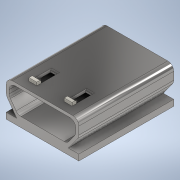
# Autodesk Inventor part: Port 3
Saved by Autodesk Inventor 2020 (Build 240168000, 168)
## iProperties
Created: 2022-11-24
Part Number: Port 3
Material: Generic
Document SubType Name: Modeling
Designer: DELL
Density: 1 g/cm^3
Appearance: Steel - Polished
Author: DELL
Autodesk Inventor part; units mm, degrees
ref_plane "YZ Plane" through (0, 0, 0) normal (1, 0, 0) x (0, 1, 0)
ref_plane "XZ Plane" through (0, 0, 0) normal (0, 1, 0) x (-1, 0, 0)
ref_plane "XY Plane" through (0, 0, 0) normal (0, 0, 1) x (1, 0, 0)
sketch "Sketch1" plane through (0, 0, 0) normal (0, 1, 0) x (-1, 0, 0)
  line L0 (0, 0) -> (0, 15.676)
  line L1 (0, 15.676) -> (-11.985, 15.676)
  line L2 (-11.985, 15.676) -> (-11.985, 0)
  line L3 (-11.985, 0) -> (0, 0)
  dimension "d1" = 15.676
  dimension "d2" = 11.985
  constraints: 8 end point, 3 perpendicular, 1 vertical
  measures "d1" distance of L0.start L0.end
  measures "d2" distance of L0.end L1.end
extrude "Extrusion1" add sketch "Sketch1" along normal blind 6
sketch "Sketch2" plane through (0, 0, 15.676) normal (0, 0, 1) x (1, 0, 0)
  line L0 (11.985, 0) -> (0, 0) projected
  line L1 (0, 0) -> (0, 6) projected
  line L2 (11.985, 0) -> (11.985, 6) projected
  line L3 (1.7246, 1) -> (10.26, 1)
  line L4 (1.7246, 1) -> (0.1886, 3.1326)
  line L5 (11.7964, 3.1326) -> (10.26, 1)
  line L6 (0, 3.717) -> (0, 5)
  line L7 (1, 6) -> (10.985, 6)
  line L8 (11.985, 5) -> (11.985, 3.7171)
  line L9 (1.7246, 1) -> (0, 1)
  line L10 (10.26, 1) -> (11.985, 1)
  arc A0 (1, 6) -> (0, 5) centre (1, 5) ccw
  arc A1 (11.985, 5) -> (10.985, 6) centre (10.985, 5) ccw
  line L11 (1, 6) -> (10.985, 6)
  line L12 (11.985, 6) -> (0, 6) projected
  arc A2 (0, 3.717) -> (0.1886, 3.1326) centre (1, 3.717) ccw
  arc A3 (11.7964, 3.1326) -> (11.985, 3.7171) centre (10.985, 3.7171) ccw
  line L13 (0, 5) -> (0.5, 5)
  arc A4 (1.5, 5.5) -> (0.5, 4.5) centre (1.5, 4.5) ccw
  line L14 (1.5, 5.5) -> (10.485, 5.5)
  arc A5 (11.485, 4.5) -> (10.485, 5.5) centre (10.485, 4.5) ccw
  line L15 (0.5, 4.5) -> (0.5, 3.8784)
  line L16 (0.6886, 3.2939) -> (1.6205, 2)
  arc A6 (0.5, 3.8784) -> (0.6886, 3.2939) centre (1.5, 3.8784) ccw
  line L17 (11.2964, 3.2939) -> (10.3641, 1.9999)
  line L18 (9.5528, 1.5845) -> (2.4319, 1.5845)
  line L19 (11.485, 4.5) -> (11.485, 3.8785)
  arc A7 (11.2964, 3.2939) -> (11.485, 3.8785) centre (10.485, 3.8785) ccw
  arc A8 (1.6205, 2) -> (2.4319, 1.5845) centre (2.4319, 2.5845) ccw
  arc A9 (9.5528, 1.5845) -> (10.3641, 1.9999) centre (9.5528, 2.5845) ccw
  line L20 (1.5, 4.5) -> (10.485, 4.5)
  line L21 (10.485, 4.5) -> (10.485, 3.8785)
  line L22 (10.485, 3.8785) -> (1.5, 3.8785)
  line L23 (1.5, 3.8785) -> (1.5, 4.5)
  line L24 (1.866, 4.5) -> (2.2834, 4.5)
  line L25 (2.2834, 4.5) -> (2.2834, 3.8785)
  line L26 (2.2834, 3.8785) -> (1.866, 3.8785)
  line L27 (1.866, 3.8785) -> (1.866, 4.5)
  line L28 (3.2834, 4.5) -> (3.2834, 3.8785)
  line L29 (2.866, 4.5) -> (3.2834, 4.5)
  line L30 (2.866, 3.8785) -> (2.866, 4.5)
  line L31 (3.2834, 3.8785) -> (2.866, 3.8785)
  line L32 (4.2834, 4.5) -> (4.2834, 3.8785)
  line L33 (3.866, 4.5) -> (4.2834, 4.5)
  line L34 (3.866, 3.8785) -> (3.866, 4.5)
  line L35 (4.2834, 3.8785) -> (3.866, 3.8785)
  line L36 (5.2834, 4.5) -> (5.2834, 3.8785)
  line L37 (4.866, 4.5) -> (5.2834, 4.5)
  line L38 (4.866, 3.8785) -> (4.866, 4.5)
  line L39 (5.2834, 3.8785) -> (4.866, 3.8785)
  line L40 (6.2834, 4.5) -> (6.2834, 3.8785)
  line L41 (5.866, 4.5) -> (6.2834, 4.5)
  line L42 (5.866, 3.8785) -> (5.866, 4.5)
  line L43 (6.2834, 3.8785) -> (5.866, 3.8785)
  line L44 (7.2834, 4.5) -> (7.2834, 3.8785)
  line L45 (6.866, 4.5) -> (7.2834, 4.5)
  line L46 (6.866, 3.8785) -> (6.866, 4.5)
  line L47 (7.2834, 3.8785) -> (6.866, 3.8785)
  line L48 (8.2834, 4.5) -> (8.2834, 3.8785)
  line L49 (7.866, 4.5) -> (8.2834, 4.5)
  line L50 (7.866, 3.8785) -> (7.866, 4.5)
  line L51 (8.2834, 3.8785) -> (7.866, 3.8785)
  line L52 (9.2834, 4.5) -> (9.2834, 3.8785)
  line L53 (8.866, 4.5) -> (9.2834, 4.5)
  line L54 (8.866, 3.8785) -> (8.866, 4.5)
  line L55 (9.2834, 3.8785) -> (8.866, 3.8785)
  line L56 (10.2834, 4.5) -> (10.2834, 3.8785)
  line L57 (9.866, 4.5) -> (10.2834, 4.5)
  line L58 (9.866, 3.8785) -> (9.866, 4.5)
  line L59 (10.2834, 3.8785) -> (9.866, 3.8785)
  line L60 (0, 6) -> (1, 6)
  line L61 (0, 6) -> (0, 5)
  line L62 (10.985, 6) -> (11.985, 6)
  line L63 (11.985, 6) -> (11.985, 5)
  line L64 (11.985, 3.7171) -> (11.985, 1)
  line L65 (0, 3.717) -> (0, 1)
  point P0 (0, 3.3944)
  point P1 (11.985, 3.3944)
  dimension "d7" = 1
  dimension "d8" = 1
  dimension "d9" = 1
  dimension "d12" = 1
  dimension "d14" = 1
  dimension "d16" = 1
  dimension "d18" = 1
  dimension "d19" = 1
  dimension "d20" = 1
  dimension "d23" = 1
  constraints: 124 end point, 21 tangent, 20 point on circle, 16 point on line, 10 centre point, 7 collinear, 6 horizontal, 4 parallel, 3 perpendicular, 1 equal radius, 1 vertical, 64 other
  measures "d7" radius of A0
  measures "d8" radius of A2
  measures "d9" radius of A3
  measures "d12" radius of A4
  measures "d14" radius of A5
  measures "d16" radius of A6
  measures "d18" radius of A7
  measures "d19" radius of A8
  measures "d20" radius of A9
  measures "d23" distance of L24.end L28.start
extrude "Extrusion2" cut sketch "Sketch2" against normal blind 16 contours L10 L5 A3 L2 | L1 A2 L4 L9 | A1 L12 L2 | L1 L12 A0
extrude "Extrusion3" cut sketch "Sketch2" against normal blind 14 contours L14 A5 L19 A7 L17 A9 L18 A8 L16 A6 L15 A4
extrude "Extrusion4" cut sketch "Sketch2" against normal blind 4 contours L20 L27 L22 L23 | L20 L30 L22 L25 | L20 L34 L22 L28 | L20 L38 L22 L32 | L20 L42 L22 L36 | L20 L46 L22 L40 | L20 L50 L22 L44 | L20 L54 L22 L48 | L20 L58 L22 L52 | L20 L21 L22 L56
extrude "Extrusion5" cut sketch "Sketch2" against normal blind 3 contours L20 L25 L22 L27 | L20 L28 L22 L30 | L20 L34 L22 L28 | L20 L32 L22 L34 | L20 L38 L22 L32 | L20 L36 L22 L38 | L20 L42 L22 L36 | L20 L40 L22 L42 | L20 L46 L22 L40 | L20 L44 L22 L46 | L20 L50 L22 L44 | L20 L48 L22 L50 | L20 L54 L22 L48 | L20 L52 L22 L54 | L20 L58 L22 L52 | L20 L56 L22 L58 | L20 L21 L22 L56
sketch "Sketch3" plane through (0, 6, 0) normal (0, 1, 0) x (1, 0, 0)
  line L0 (2.4319, -10.8223) -> (2.4319, -13.627)
  line L1 (2.4319, -15.676) -> (2.4319, -1.676) projected
  line L2 (2.4319, -10.8223) -> (2.4319, -13.627)
  line L3 (2.4319, -13.627) -> (3.7319, -13.627)
  line L4 (3.7319, -13.627) -> (3.7319, -10.8223)
  line L5 (3.7319, -10.8223) -> (2.4319, -10.8223)
  line L6 (9.5528, -15.676) -> (9.5528, -1.676) projected
  line L7 (9.5528, -10.8223) -> (9.5528, -13.627)
  line L8 (9.5528, -13.627) -> (8.2528, -13.627)
  line L9 (8.2528, -13.627) -> (8.2528, -10.8223)
  line L10 (8.2528, -10.8223) -> (9.5528, -10.8223)
  line L11 (2.4319, -13.627) -> (3.7319, -13.627)
  line L12 (3.7319, -13.627) -> (3.7319, -14.3676)
  line L13 (3.7319, -14.3676) -> (2.4319, -14.3676)
  line L14 (2.4319, -14.3676) -> (2.4319, -13.627)
  line L15 (8.2528, -13.627) -> (9.5528, -13.627)
  line L16 (9.5528, -13.627) -> (9.5528, -14.3676)
  line L17 (9.5528, -14.3676) -> (8.2528, -14.3676)
  line L18 (8.2528, -14.3676) -> (8.2528, -13.627)
  point P0 (0, 0)
  dimension "d38" = 1.3
  dimension "d40" = 1.3
  constraints: 34 end point, 7 perpendicular, 6 equal length, 4 point on line, 2 horizontal
  measures "d38" distance of L0.end L3.end
  measures "d40" distance of L7.end L8.end
extrude "Extrusion6" cut sketch "Sketch3" against normal blind 1 contours L5 L4 L3 L0 | L8 L9 L10 L6
extrude "Extrusion7" add sketch "Sketch3" along normal blind 0.5 contours L3 L12 L13 L1 | L17 L18 L8 L6
chamfer "Chamfer1" distance 0.2 angle 45 3 edges at (1.5, 4.1892, 11.676) (10.485, 4.1892, 11.676) (8.9028, 6.5, 13.627)
chamfer "Chamfer2" distance 0.2 angle 45 1 edges at (3.0819, 6.5, 13.627)
chamfer "Chamfer3" distance 0.2 angle 45 2 edges at (3.0819, 6, 10.8223) (8.9028, 6, 10.8223)
body "Solid1"
